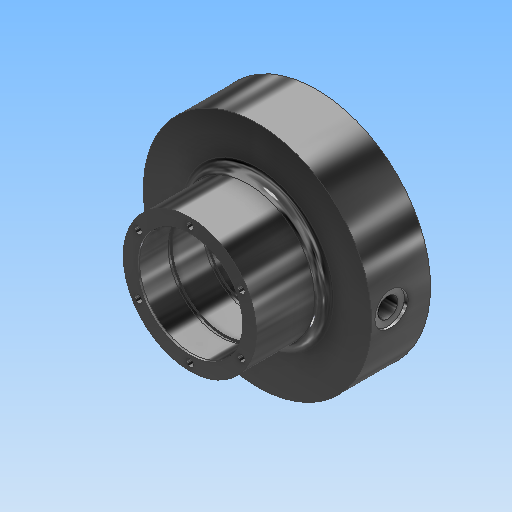
# Autodesk Inventor part: 7055-193 PART1
Saved by Autodesk Inventor 2020.1 (Build 241239000, 239)
## iProperties
Created: 2001-03-07
Part Number: 7055-193 PART1
Document SubType Name: Modeling
Designer: Joe M
Material: Steel, Mild
Engineer: Joe M
Density: 7.86 g/cm^3
Appearance: Chrome - Polished Black
Control State: 0
Master: False
Checked Out: False
Shininess: 20.0
Length Units: 11269
Angle Units: 11279
Time Units: 11290
Mass Units: 11283
Length Display Precision: 3
Angle Display Precision: 2
Compacted: True
Density: 0.0
Volumn: 0.0
Area: 0.0
PropertySet Name: Model Information
Author: Joe M
Autodesk Inventor part; units mm, degrees
ref_plane "WorkPlane4" through (-200.4653, -160.3265, -69.5) normal (1, 0, 0) x (0, 1, 0)
ref_plane "WorkPlane6" through (149.5347, -160.3265, -69.5) normal (1, 0, 0) x (0, 1, 0)
sketch "Sketch1" plane through (-200.4653, -160.3265, -69.5) normal (0, 0, 1) x (1, 0, 0)
  circle A0 centre (200.4653, 160.3265) radius 120
  dimension "d76" = 240
  constraints: 1 centre point, 1 other
  measures "d76" diameter of A0
extrude "ExtrusionBlind1" add sketch "Sketch1" along normal blind 139
ref_plane "WorkPlane7" through (120, 0, -69.5) normal (1, 0, 0) x (0, 1, 0)
ref_plane "WorkPlane1" through (0, 0, 35.425) normal (0, 0, 1) x (1, 0, 0)
ref_plane "WorkPlane9" through (0, 0, -69.5) normal (-0.001, -1, 0) x (1, -0.001, 0)
ref_plane "WorkPlane2" through (0, 0, -0.575) normal (0, 0, 1) x (1, 0, 0)
sketch "Sketch2" plane through (0, 0, 69.5) normal (0, 0, 1) x (1, 0, 0)
  point P0 (0, 62.5)
ref_plane "WorkPlane10" through (119.9999, -0.1181, -69.5) normal (1, -0.001, 0) x (0.001, 1, 0)
sketch "Sketch3" plane through (0, 0, 69.5) normal (0, 0, 1) x (1, 0, 0)
  circle A0 centre (0, 0) radius 55
  circle A1 centre (0, 0) radius 120 projected
  dimension "d77" = 110
  constraints: 1 centre point, 1 concentric
  measures "d77" diameter of A0
extrude "ExtrusionThru1" cut sketch "Sketch3" against normal through all contours A0
ref_plane "WorkPlane3" through (0, 0, -27.575) normal (0, 0, 1) x (1, 0, 0)
sketch "Sketch4" plane through (119.9999, -0.1181, -69.5) normal (1, -0.001, 0) x (0.001, 1, 0)
  point P0 (0, 47)
chamfer "Chamfer1" distance 2 angle 15 1 edges at (-55, 0, 69.5) measured on face at (-51.6831, -18.8111, -23.1667)
sketch "Sketch5" plane through (0, 0, 35.425) normal (0, 0, 1) x (1, 0, 0)
  circle A0 centre (0, 0) radius 57
  circle A1 centre (0, 0) radius 55.5359 projected
  dimension "d78" = 114
  constraints: 1 centre point, 1 concentric
  measures "d78" diameter of A0
extrude "ExtrusionMidplane1" cut sketch "Sketch5" along normal mid plane 4.15 contours A0 | A1
sketch "Sketch6" plane through (0, 0, -0.575) normal (0, 0, 1) x (1, 0, 0)
  circle A0 centre (0, 0) radius 57
  circle A1 centre (0, 0) radius 55.5359 projected
  dimension "d79" = 114
  constraints: 1 centre point, 1 concentric
  measures "d79" diameter of A0
extrude "ExtrusionMidplane2" cut sketch "Sketch6" along normal mid plane 4.15 contours A0 | A1
sketch "Sketch7" plane through (0, 0, -27.575) normal (0, 0, 1) x (1, 0, 0)
  circle A0 centre (0, 0) radius 57
  circle A1 centre (0, 0) radius 55.5359 projected
  dimension "d80" = 114
  constraints: 1 centre point, 1 concentric
  measures "d80" diameter of A0
extrude "ExtrusionMidplane3" cut sketch "Sketch7" along normal mid plane 4.15 contours A0 | A1
sketch "Sketch8" plane through (0, 0, -69.5) normal (0, 0, -1) x (-1, 0, 0)
  circle A0 centre (0, 0) radius 72.5
  circle A1 centre (0, 0) radius 120 projected
  dimension "d81" = 145
  constraints: 1 centre point, 1 concentric
  measures "d81" diameter of A0
extrude "ExtrusionBlind2" cut sketch "Sketch8" against normal blind 5 contours A0
sketch "Sketch9" plane through (0, 0, -64.5) normal (0, 0, -1) x (-1, 0, 0)
  point P0 (0, 0)
hole "AM_HOLE_UCnsk_1" at (0, 0, -64.5) direction (0, 0, 1) diameter 110 depth 34.85 countersink diameter 145 countersink angle 90
hole "Hole1" at (0, 62.5, 69.5) direction (0, 0, -1) diameter 8 depth 20 tip angle 118
pattern_circular "PolarArray1" count 6 over 360 about axis through (0, 0, 69.5) along (0, 0, 1) of "Hole1"
sketch "Sketch13" plane through (0, 0, -69.5) normal (0, 0, -1) x (-1, 0, 0)
  circle A0 centre (0, 0) radius 80
  circle A1 centre (0, 0) radius 135.6604
  circle A2 centre (0, 0) radius 120 projected
  dimension "d82" = 271.3209
  dimension "d83" = 160
  constraints: 2 centre point, 1 coincident, 1 concentric
  measures "d82" diameter of A1
  measures "d83" diameter of A0
extrude "ExtrusionBlind3" cut sketch "Sketch13" against normal blind 6 contours A1 | A2
ref_plane "WorkPlane5" through (0, 0, -22.5) normal (0, 0, -1) x (-1, 0, 0)
ref_plane "WorkPlane8" through (0, 0, -22.5) normal (0, 0, -1) x (-1, 0, 0)
sketch "Sketch14" plane through (0, 0, -63.5) normal (0, 0, -1) x (-1, 0, 0)
  point P0 (101.4222, 27.176)
hole "Hole2" at (-101.4222, 27.176, -63.5) direction (0, 0, 1) diameter 9.85 depth 20 tip angle 118
sketch "Sketch16" plane through (0, 0, -22.5) normal (0, 0, -1) x (-1, 0, 0)
  point P0 (-120, 0)
pattern_circular "PolarArray2" count 12 over 360 about axis through (0, 0, 69.5) along (0, 0, -1) of "Hole2"
sketch "Sketch18" plane through (0, 0, 69.5) normal (0, 0, 1) x (1, 0, 0)
  circle A0 centre (0, 0) radius 70
  circle A1 centre (0, 0) radius 138.6706
  circle A2 centre (0, 0) radius 120 projected
  dimension "d84" = 277.3413
  dimension "d85" = 140
  constraints: 2 centre point, 1 coincident, 1 concentric
  measures "d84" diameter of A1
  measures "d85" diameter of A0
extrude "ExtrusionBlind4" cut sketch "Sketch18" against normal blind 71 contours A1 | A2
fillet "Fillet1" radius 10 1 edges at (-70, 0, -1.5)
sketch "Sketch20" plane through (-200.4653, -160.3265, -69.5) normal (1, 0, 0) x (0, 1, 0)
  line L0 (71.3265, 37) -> (71.3265, 56)
  line L1 (71.3265, 37) -> (40.3265, 37)
  line L2 (40.3265, 56) -> (40.3265, 37)
  line L3 (71.3265, 56) -> (40.3265, 56)
  line L4 (40.3265, 68) -> (280.3265, 68) projected
  dimension "d88" = 31
  dimension "d89" = 19
  dimension "d91" = 12
  constraints: 8 end point, 2 horizontal, 2 vertical
  measures "d88" distance between parallel lines of L0 L2
  measures "d89" distance between parallel lines of L3 L1
  measures "d91" distance between parallel lines of L4 L3
extrude "ExtrusionThru3" [suppressed]
sketch "Sketch21" plane through (120, 0, -69.5) normal (1, 0, 0) x (0, 1, 0)
  circle A0 centre (0, 47) radius 17.5
  line L0 (-120, 68) -> (120, 68) projected
  dimension "d90" = 35
  dimension "d96" = 21
  constraints: 1 centre point
  measures "d90" diameter of A0
  measures "d96" distance from line of L0 A0.centre
extrude "ExtrusionBlind5" cut sketch "Sketch21" against normal blind 4
hole "Hole3" at (119.9999, -0.1181, -22.5) direction (-1, 0.001, 0) diameter 21 depth 44.4 tip angle 118
mirror "Mirror1" about plane through (0, 0, 0) normal (1, 0, 0) of "ExtrusionBlind5", "Hole3"
body "Solid1"
